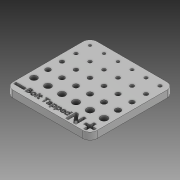
# Autodesk Inventor part: Tapped Test Print
Saved by Autodesk Inventor 2022 (Build 260153000, 153)
## iProperties
Created: 2022-01-18
Part Number: Tapped Test Print
Material: ABS Plastic
Document SubType Name: Modeling
Density: 1.06 g/cm^3
Appearance: Smooth - Medium Gray
Autodesk Inventor part; units mm, degrees
ref_plane "YZ Plane" through (0, 0, 0) normal (1, 0, 0) x (0, 1, 0)
ref_plane "XZ Plane" through (0, 0, 0) normal (0, 1, 0) x (-1, 0, 0)
ref_plane "XY Plane" through (0, 0, 0) normal (0, 0, 1) x (1, 0, 0)
sketch "Sketch1" plane through (0, 0, 0) normal (0, 1, 0) x (-1, 0, 0)
  circle A0 centre (0, 12.7) radius 1.4986
  circle A1 centre (-12.7, 12.7) radius 1.5621
  circle A2 centre (-25.4, 12.7) radius 1.6256
  circle A3 centre (-38.1, 12.7) radius 1.6891
  circle A4 centre (-50.8, 12.7) radius 1.7526
  circle A5 centre (0, 25.4) radius 1.8288
  circle A6 centre (-12.7, 25.4) radius 1.8923
  circle A7 centre (-25.4, 25.4) radius 1.9558
  circle A8 centre (-38.1, 25.4) radius 2.0193
  circle A9 centre (-50.8, 25.4) radius 2.0828
  circle A10 centre (0, 38.1) radius 2.2352
  circle A11 centre (-12.7, 38.1) radius 2.2987
  circle A12 centre (-25.4, 38.1) radius 2.3622
  circle A13 centre (-38.1, 38.1) radius 2.4257
  circle A14 centre (-50.8, 38.1) radius 2.4892
  line L0 (4.7625, 64.6906) -> (-4.7625, 64.6906)
  line L1 (-4.7625, 64.6906) -> (-4.7625, 62.3094)
  line L2 (-4.7625, 62.3094) -> (4.7625, 62.3094)
  line L3 (4.7625, 62.3094) -> (4.7625, 64.6906)
  line L4 (4.7625, 64.6906) -> (-4.7625, 62.3094) construction
  line L5 (-4.7625, 64.6906) -> (4.7625, 62.3094) construction
  line L6 (-58.7375, 64.6906) -> (-68.2625, 64.6906)
  line L7 (-68.2625, 64.6906) -> (-68.2625, 62.3094)
  line L8 (-68.2625, 62.3094) -> (-58.7375, 62.3094)
  line L9 (-58.7375, 62.3094) -> (-58.7375, 64.6906)
  line L10 (-58.7375, 64.6906) -> (-68.2625, 62.3094) construction
  line L11 (-68.2625, 64.6906) -> (-58.7375, 62.3094) construction
  line L12 (-64.6906, 58.7375) -> (-62.3094, 58.7375)
  line L13 (-62.3094, 58.7375) -> (-62.3094, 68.2625)
  line L14 (-62.3094, 68.2625) -> (-64.6906, 68.2625)
  line L15 (-64.6906, 68.2625) -> (-64.6906, 58.7375)
  line L16 (-64.6906, 58.7375) -> (-62.3094, 68.2625) construction
  line L17 (-62.3094, 58.7375) -> (-64.6906, 68.2625) construction
  circle A15 centre (-63.5, 38.1) radius 2.5527
  circle A16 centre (-63.5, 25.4) radius 2.1463
  circle A17 centre (-63.5, 12.7) radius 1.8161
  circle A18 centre (0, 0) radius 1.1684
  circle A19 centre (-12.7, 0) radius 1.2319
  circle A20 centre (-25.4, 0) radius 1.2954
  circle A21 centre (-38.1, 0) radius 1.3589
  circle A22 centre (-50.8, 0) radius 1.4224
  circle A23 centre (-63.5, 0) radius 1.4859
  line L18 (-46.0375, 68.2625) -> (-46.0375, 58.7375)
  line L19 (-46.0375, 58.7375) -> (-48.4188, 58.7375)
  line L20 (-48.4188, 58.7375) -> (-53.1813, 64.5177)
  line L21 (-53.1813, 64.5177) -> (-53.1813, 58.7375)
  line L22 (-53.1813, 58.7375) -> (-55.5625, 58.7375)
  line L23 (-55.5625, 58.7375) -> (-55.5625, 68.2625)
  line L24 (-55.5625, 68.2625) -> (-53.1813, 68.2625)
  line L25 (-53.1813, 68.2625) -> (-48.4188, 62.4823)
  line L26 (-48.4188, 62.4823) -> (-48.4188, 68.2625)
  line L27 (-48.4188, 68.2625) -> (-46.0375, 68.2625)
  line L28 (-50.8, 65.3724) -> (-50.8, 61.6276) construction
  line L29 (6.35, -6.35) -> (-69.85, -6.35)
  line L30 (-69.85, -6.35) -> (-69.85, 69.85)
  line L31 (-69.85, 69.85) -> (6.35, 69.85)
  line L32 (6.35, 69.85) -> (6.35, -6.35)
  line L33 (6.35, -6.35) -> (-69.85, 69.85) construction
  line L34 (-69.85, -6.35) -> (6.35, 69.85) construction
  circle A24 centre (-12.7, 50.8) radius 2.9845
  circle A25 centre (-25.4, 50.8) radius 3.048
  circle A26 centre (-38.1, 50.8) radius 3.1115
  circle A27 centre (-50.8, 50.8) radius 3.175
  circle A28 centre (-63.5, 50.8) radius 3.2385
  circle A29 centre (0, 50.8) radius 2.921
  line L35 (0, 73.2249) -> (-50.8, 73.2249) construction
  line L36 (-50.8, 73.2249) -> (-50.8, 53.7751) construction
  line L37 (-50.8, 53.7751) -> (0, 53.7751) construction
  line L38 (0, 53.7751) -> (0, 73.2249) construction
  spline S0 degree 2 poles (-9.9909, 63.8715) (-9.9909, 64.2275) (-9.72, 64.7654) (-9.4956, 64.9434) knots 0 0 0 1 2 2 2
  spline S1 degree 2 poles (-9.4956, 64.9434) (-9.2247, 65.1562) (-8.5823, 65.3342) (-8.0831, 65.3342) knots 0 0 0 1 2 2 2
  line L39 (-8.0831, 65.3342) -> (-6.1754, 65.3342)
  line L40 (-6.1754, 65.3342) -> (-6.1754, 60.559)
  line L41 (-6.1754, 60.559) -> (-7.8587, 60.559)
  spline S2 degree 2 poles (-7.8587, 60.559) (-8.385, 60.559) (-8.9267, 60.6403) (-9.1628, 60.768) knots 0 0 0 1 2 2 2
  spline S3 degree 2 poles (-9.1628, 60.768) (-9.422, 60.9034) (-9.6736, 61.3678) (-9.6736, 61.6696) knots 0 0 0 1 2 2 2
  spline S4 degree 2 poles (-9.6736, 61.6696) (-9.6736, 62.0179) (-9.3253, 62.5635) (-9.0157, 62.6912) knots 0 0 0 1 2 2 2
  line L42 (-9.0157, 62.6912) -> (-9.0157, 62.7145)
  spline S5 degree 2 poles (-9.0157, 62.7145) (-9.4607, 62.8073) (-9.9909, 63.3839) (-9.9909, 63.8715) knots 0 0 0 1 2 2 2
  spline S6 degree 2 poles (-8.7526, 63.8521) (-8.7526, 63.6277) (-8.5746, 63.3762) (-8.3966, 63.3104) knots 0 0 0 1 2 2 2
  spline S7 degree 2 poles (-8.3966, 63.3104) (-8.2882, 63.2678) (-7.9051, 63.2601) (-7.5878, 63.2601) knots 0 0 0 1 2 2 2
  line L43 (-7.5878, 63.2601) -> (-7.3672, 63.2601)
  line L44 (-7.3672, 63.2601) -> (-7.3672, 64.4636)
  line L45 (-7.3672, 64.4636) -> (-7.433, 64.4636)
  spline S8 degree 2 poles (-7.433, 64.4636) (-7.8974, 64.4636) (-8.2534, 64.4519) (-8.4391, 64.3707) knots 0 0 0 1 2 2 2
  spline S9 degree 2 poles (-8.4391, 64.3707) (-8.6017, 64.2972) (-8.7526, 64.0263) (-8.7526, 63.8521) knots 0 0 0 1 2 2 2
  spline S10 degree 2 poles (-8.4546, 61.9057) (-8.4546, 61.7896) (-8.3347, 61.5458) (-8.2108, 61.4916) knots 0 0 0 1 2 2 2
  spline S11 degree 2 poles (-8.2108, 61.4916) (-8.0947, 61.4375) (-7.7697, 61.4297) (-7.4485, 61.4297) knots 0 0 0 1 2 2 2
  line L46 (-7.4485, 61.4297) -> (-7.3672, 61.4297)
  line L47 (-7.3672, 61.4297) -> (-7.3672, 62.4436)
  line L48 (-7.3672, 62.4436) -> (-7.5182, 62.4436)
  spline S12 degree 2 poles (-7.5182, 62.4436) (-7.8239, 62.4436) (-8.0715, 62.432) (-8.2031, 62.37) knots 0 0 0 1 2 2 2
  spline S13 degree 2 poles (-8.2031, 62.37) (-8.3463, 62.3004) (-8.4546, 62.0643) (-8.4546, 61.9057) knots 0 0 0 1 2 2 2
  spline S14 degree 2 poles (-14.0695, 63.5348) (-14.0695, 64.4249) (-13.0982, 65.4465) (-12.2121, 65.4465) knots 0 0 0 1 2 2 2
  spline S15 degree 2 poles (-12.2121, 65.4465) (-11.3298, 65.4465) (-10.3508, 64.4249) (-10.3508, 63.5348) knots 0 0 0 1 2 2 2
  spline S16 degree 2 poles (-10.3508, 63.5348) (-10.3508, 62.6371) (-11.3298, 61.6193) (-12.2121, 61.6193) knots 0 0 0 1 2 2 2
  spline S17 degree 2 poles (-12.2121, 61.6193) (-13.0944, 61.6193) (-14.0695, 62.6409) (-14.0695, 63.5348) knots 0 0 0 1 2 2 2
  spline S18 degree 2 poles (-12.9202, 63.5426) (-12.9202, 63.2214) (-12.8158, 62.7918) (-12.7229, 62.6641) knots 0 0 0 1 2 2 2
  spline S19 degree 2 poles (-12.7229, 62.6641) (-12.6223, 62.5287) (-12.3707, 62.4242) (-12.2121, 62.4242) knots 0 0 0 1 2 2 2
  spline S20 degree 2 poles (-12.2121, 62.4242) (-12.0573, 62.4242) (-11.8135, 62.5171) (-11.7129, 62.6487) knots 0 0 0 1 2 2 2
  spline S21 degree 2 poles (-11.7129, 62.6487) (-11.6162, 62.7725) (-11.5001, 63.2098) (-11.5001, 63.5426) knots 0 0 0 1 2 2 2
  spline S22 degree 2 poles (-11.5001, 63.5426) (-11.5001, 63.8715) (-11.6084, 64.2778) (-11.6974, 64.4016) knots 0 0 0 1 2 2 2
  spline S23 degree 2 poles (-11.6974, 64.4016) (-11.7864, 64.5255) (-12.0573, 64.6416) (-12.2198, 64.6416) knots 0 0 0 1 2 2 2
  spline S24 degree 2 poles (-12.2198, 64.6416) (-12.3553, 64.6416) (-12.6339, 64.5255) (-12.719, 64.4094) knots 0 0 0 1 2 2 2
  spline S25 degree 2 poles (-12.719, 64.4094) (-12.8158, 64.2739) (-12.9202, 63.8831) (-12.9202, 63.5426) knots 0 0 0 1 2 2 2
  line L49 (-15.7877, 65.3342) -> (-14.6655, 65.3342)
  line L50 (-14.6655, 65.3342) -> (-14.6655, 60.3462)
  line L51 (-14.6655, 60.3462) -> (-15.7877, 60.3462)
  line L52 (-15.7877, 60.3462) -> (-15.7877, 65.3342)
  spline S26 degree 2 poles (-18.0244, 65.4039) (-17.3394, 65.4039) (-16.7125, 64.8389) (-16.7125, 64.1965) knots 0 0 0 1 2 2 2
  line L53 (-16.7125, 64.1965) -> (-16.7125, 62.5132)
  line L54 (-16.7125, 62.5132) -> (-16.283, 62.5132)
  line L55 (-16.283, 62.5132) -> (-16.283, 61.7316)
  line L56 (-16.283, 61.7316) -> (-16.7125, 61.7316)
  line L57 (-16.7125, 61.7316) -> (-16.7125, 60.7022)
  line L58 (-16.7125, 60.7022) -> (-17.8348, 60.7022)
  line L59 (-17.8348, 60.7022) -> (-17.8348, 61.7316)
  line L60 (-17.8348, 61.7316) -> (-18.9183, 61.7316)
  line L61 (-18.9183, 61.7316) -> (-18.9183, 62.5132)
  line L62 (-18.9183, 62.5132) -> (-17.8348, 62.5132)
  line L63 (-17.8348, 62.5132) -> (-17.8348, 63.7941)
  spline S27 degree 2 poles (-17.8348, 63.7941) (-17.8348, 63.9837) (-17.8425, 64.2662) (-17.8889, 64.3784) knots 0 0 0 1 2 2 2
  spline S28 degree 2 poles (-17.8889, 64.3784) (-17.9354, 64.4906) (-18.1637, 64.6222) (-18.3804, 64.6222) knots 0 0 0 1 2 2 2
  spline S29 degree 2 poles (-18.3804, 64.6222) (-18.4733, 64.6222) (-18.7635, 64.5448) (-18.8215, 64.5139) knots 0 0 0 1 2 2 2
  line L64 (-18.8215, 64.5139) -> (-18.9183, 64.5139)
  line L65 (-18.9183, 64.5139) -> (-18.9183, 65.3033)
  spline S30 degree 2 poles (-18.9183, 65.3033) (-18.7364, 65.3497) (-18.3262, 65.4039) (-18.0244, 65.4039) knots 0 0 0 1 2 2 2
  line L66 (-22.281, 65.3342) -> (-22.281, 61.4684)
  line L67 (-22.281, 61.4684) -> (-20.8686, 61.4684)
  line L68 (-20.8686, 61.4684) -> (-20.8686, 60.559)
  line L69 (-20.8686, 60.559) -> (-24.8931, 60.559)
  line L70 (-24.8931, 60.559) -> (-24.8931, 61.4684)
  line L71 (-24.8931, 61.4684) -> (-23.4806, 61.4684)
  line L72 (-23.4806, 61.4684) -> (-23.4806, 65.3342)
  line L73 (-23.4806, 65.3342) -> (-22.281, 65.3342)
  spline S31 degree 2 poles (-27.3039, 64.9511) (-27.1878, 65.0479) (-27.0059, 65.2027) (-26.8511, 65.2801) knots 0 0 0 1 2 2 2
  spline S32 degree 2 poles (-26.8511, 65.2801) (-26.7002, 65.3536) (-26.4139, 65.431) (-26.1585, 65.431) knots 0 0 0 1 2 2 2
  spline S33 degree 2 poles (-26.1585, 65.431) (-25.6786, 65.431) (-25.0479, 64.7886) (-25.0479, 64.301) knots 0 0 0 1 2 2 2
  spline S34 degree 2 poles (-25.0479, 64.301) (-25.0479, 63.9024) (-25.369, 63.4071) (-25.6709, 63.2639) knots 0 0 0 1 2 2 2
  spline S35 degree 2 poles (-25.6709, 63.2639) (-25.9766, 63.1169) (-26.824, 63.0008) (-27.3116, 62.9699) knots 0 0 0 1 2 2 2
  line L74 (-27.3116, 62.9699) -> (-27.3116, 62.9505)
  spline S36 degree 2 poles (-27.3116, 62.9505) (-27.3116, 62.6525) (-26.8705, 62.4242) (-26.4293, 62.4242) knots 0 0 0 1 2 2 2
  spline S37 degree 2 poles (-26.4293, 62.4242) (-26.232, 62.4242) (-25.698, 62.5674) (-25.4464, 62.6796) knots 0 0 0 1 2 2 2
  line L75 (-25.4464, 62.6796) -> (-25.3497, 62.6796)
  line L76 (-25.3497, 62.6796) -> (-25.3497, 61.8089)
  spline S38 degree 2 poles (-25.3497, 61.8089) (-25.5161, 61.7625) (-26.2591, 61.6309) (-26.6383, 61.6309) knots 0 0 0 1 2 2 2
  spline S39 degree 2 poles (-26.6383, 61.6309) (-27.567, 61.6309) (-28.4184, 62.2501) (-28.4184, 62.8847) knots 0 0 0 1 2 2 2
  line L77 (-28.4184, 62.8847) -> (-28.4184, 65.3342)
  line L78 (-28.4184, 65.3342) -> (-27.3039, 65.3342)
  line L79 (-27.3039, 65.3342) -> (-27.3039, 64.9511)
  line L80 (-27.3039, 64.3939) -> (-27.3039, 63.647)
  spline S40 degree 2 poles (-27.3039, 63.647) (-27.0175, 63.6741) (-26.6654, 63.7167) (-26.4951, 63.7786) knots 0 0 0 1 2 2 2
  spline S41 degree 2 poles (-26.4951, 63.7786) (-26.3442, 63.8289) (-26.1817, 64.0379) (-26.1817, 64.2082) knots 0 0 0 1 2 2 2
  spline S42 degree 2 poles (-26.1817, 64.2082) (-26.1817, 64.4597) (-26.4564, 64.6493) (-26.7234, 64.6493) knots 0 0 0 1 2 2 2
  spline S43 degree 2 poles (-26.7234, 64.6493) (-26.8705, 64.6493) (-27.1801, 64.5139) (-27.3039, 64.3939) knots 0 0 0 1 2 2 2
  spline S44 degree 2 poles (-32.7795, 63.4845) (-32.7795, 64.3475) (-31.905, 65.4039) (-31.2626, 65.4039) knots 0 0 0 1 2 2 2
  spline S45 degree 2 poles (-31.2626, 65.4039) (-30.9956, 65.4039) (-30.597, 65.2839) (-30.3726, 65.1524) knots 0 0 0 1 2 2 2
  line L81 (-30.3726, 65.1524) -> (-30.3726, 66.6538)
  line L82 (-30.3726, 66.6538) -> (-29.2503, 66.6538)
  line L83 (-29.2503, 66.6538) -> (-29.2503, 61.7316)
  line L84 (-29.2503, 61.7316) -> (-30.3726, 61.7316)
  line L85 (-30.3726, 61.7316) -> (-30.3726, 62.1108)
  spline S46 degree 2 poles (-30.3726, 62.1108) (-30.6202, 61.8979) (-31.131, 61.6348) (-31.4677, 61.6348) knots 0 0 0 1 2 2 2
  spline S47 degree 2 poles (-31.4677, 61.6348) (-32.0946, 61.6348) (-32.7795, 62.6293) (-32.7795, 63.4845) knots 0 0 0 1 2 2 2
  spline S48 degree 2 poles (-31.6302, 63.5077) (-31.6302, 62.9815) (-31.3052, 62.5094) (-30.9646, 62.5094) knots 0 0 0 1 2 2 2
  spline S49 degree 2 poles (-30.9646, 62.5094) (-30.8137, 62.5094) (-30.5157, 62.6061) (-30.3726, 62.7028) knots 0 0 0 1 2 2 2
  line L86 (-30.3726, 62.7028) -> (-30.3726, 64.51)
  spline S50 degree 2 poles (-30.3726, 64.51) (-30.4616, 64.5487) (-30.6783, 64.5796) (-30.8253, 64.5796) knots 0 0 0 1 2 2 2
  spline S51 degree 2 poles (-30.8253, 64.5796) (-31.2316, 64.5796) (-31.6302, 64.0456) (-31.6302, 63.5077) knots 0 0 0 1 2 2 2
  spline S52 degree 2 poles (-36.9123, 63.4845) (-36.9123, 64.3475) (-36.0378, 65.4039) (-35.3954, 65.4039) knots 0 0 0 1 2 2 2
  spline S53 degree 2 poles (-35.3954, 65.4039) (-35.1284, 65.4039) (-34.7298, 65.2839) (-34.5054, 65.1524) knots 0 0 0 1 2 2 2
  line L87 (-34.5054, 65.1524) -> (-34.5054, 66.6538)
  line L88 (-34.5054, 66.6538) -> (-33.3832, 66.6538)
  line L89 (-33.3832, 66.6538) -> (-33.3832, 61.7316)
  line L90 (-33.3832, 61.7316) -> (-34.5054, 61.7316)
  line L91 (-34.5054, 61.7316) -> (-34.5054, 62.1108)
  spline S54 degree 2 poles (-34.5054, 62.1108) (-34.753, 61.8979) (-35.2638, 61.6348) (-35.6005, 61.6348) knots 0 0 0 1 2 2 2
  spline S55 degree 2 poles (-35.6005, 61.6348) (-36.2274, 61.6348) (-36.9123, 62.6293) (-36.9123, 63.4845) knots 0 0 0 1 2 2 2
  spline S56 degree 2 poles (-35.763, 63.5077) (-35.763, 62.9815) (-35.438, 62.5094) (-35.0974, 62.5094) knots 0 0 0 1 2 2 2
  spline S57 degree 2 poles (-35.0974, 62.5094) (-34.9465, 62.5094) (-34.6486, 62.6061) (-34.5054, 62.7028) knots 0 0 0 1 2 2 2
  line L92 (-34.5054, 62.7028) -> (-34.5054, 64.51)
  spline S58 degree 2 poles (-34.5054, 64.51) (-34.5944, 64.5487) (-34.8111, 64.5796) (-34.9581, 64.5796) knots 0 0 0 1 2 2 2
  spline S59 degree 2 poles (-34.9581, 64.5796) (-35.3645, 64.5796) (-35.763, 64.0456) (-35.763, 63.5077) knots 0 0 0 1 2 2 2
  spline S60 degree 2 poles (-39.3618, 65.431) (-38.3403, 65.431) (-37.2529, 64.4558) (-37.2529, 63.5542) knots 0 0 0 1 2 2 2
  spline S61 degree 2 poles (-37.2529, 63.5542) (-37.2529, 62.6719) (-38.2667, 61.6193) (-39.18, 61.6193) knots 0 0 0 1 2 2 2
  spline S62 degree 2 poles (-39.18, 61.6193) (-40.0042, 61.6193) (-40.8401, 62.5132) (-40.8401, 63.3413) knots 0 0 0 1 2 2 2
  line L93 (-40.8401, 63.3413) -> (-40.8401, 63.7477)
  line L94 (-40.8401, 63.7477) -> (-38.3751, 63.7477)
  spline S63 degree 2 poles (-38.3751, 63.7477) (-38.3906, 63.9992) (-38.5724, 64.332) (-38.7195, 64.4326) knots 0 0 0 1 2 2 2
  spline S64 degree 2 poles (-38.7195, 64.4326) (-38.8627, 64.5332) (-39.2496, 64.6183) (-39.4779, 64.6183) knots 0 0 0 1 2 2 2
  spline S65 degree 2 poles (-39.4779, 64.6183) (-39.6714, 64.6183) (-40.0507, 64.5332) (-40.2093, 64.4597) knots 0 0 0 1 2 2 2
  spline S66 degree 2 poles (-40.2093, 64.4597) (-40.3486, 64.4016) (-40.5808, 64.2585) (-40.6543, 64.2043) knots 0 0 0 1 2 2 2
  line L95 (-40.6543, 64.2043) -> (-40.7743, 64.2043)
  line L96 (-40.7743, 64.2043) -> (-40.7743, 65.133)
  spline S67 degree 2 poles (-40.7743, 65.133) (-40.635, 65.1872) (-40.4105, 65.2801) (-40.2093, 65.3265) knots 0 0 0 1 2 2 2
  spline S68 degree 2 poles (-40.2093, 65.3265) (-40.0274, 65.3768) (-39.6405, 65.431) (-39.3618, 65.431) knots 0 0 0 1 2 2 2
  spline S69 degree 2 poles (-39.7333, 63.0705) (-39.7256, 62.7145) (-39.4122, 62.3391) (-39.091, 62.3391) knots 0 0 0 1 2 2 2
  spline S70 degree 2 poles (-39.091, 62.3391) (-38.762, 62.3391) (-38.3906, 62.7338) (-38.3712, 63.0705) knots 0 0 0 1 2 2 2
  line L97 (-38.3712, 63.0705) -> (-39.7333, 63.0705)
  line L98 (-44.6904, 65.3342) -> (-43.5682, 65.3342)
  line L99 (-43.5682, 65.3342) -> (-43.5682, 64.9589)
  spline S71 degree 2 poles (-43.5682, 64.9589) (-43.4599, 65.0479) (-43.1812, 65.253) (-43.0729, 65.3071) knots 0 0 0 1 2 2 2
  spline S72 degree 2 poles (-43.0729, 65.3071) (-42.9413, 65.3691) (-42.6782, 65.4348) (-42.4963, 65.4348) knots 0 0 0 1 2 2 2
  spline S73 degree 2 poles (-42.4963, 65.4348) (-41.881, 65.4348) (-41.1613, 64.4132) (-41.1613, 63.5619) knots 0 0 0 1 2 2 2
  spline S74 degree 2 poles (-41.1613, 63.5619) (-41.1613, 63.0898) (-41.405, 62.3971) (-41.6179, 62.1417) knots 0 0 0 1 2 2 2
  spline S75 degree 2 poles (-41.6179, 62.1417) (-41.8152, 61.9057) (-42.3725, 61.6348) (-42.682, 61.6348) knots 0 0 0 1 2 2 2
  spline S76 degree 2 poles (-42.682, 61.6348) (-42.9645, 61.6348) (-43.3283, 61.7548) (-43.5682, 61.8786) knots 0 0 0 1 2 2 2
  line L100 (-43.5682, 61.8786) -> (-43.5682, 60.3462)
  line L101 (-43.5682, 60.3462) -> (-44.6904, 60.3462)
  line L102 (-44.6904, 60.3462) -> (-44.6904, 65.3342)
  line L103 (-43.5682, 64.3436) -> (-43.5682, 62.5751)
  spline S77 degree 2 poles (-43.5682, 62.5751) (-43.4869, 62.5326) (-43.2161, 62.4784) (-43.1193, 62.4784) knots 0 0 0 1 2 2 2
  spline S78 degree 2 poles (-43.1193, 62.4784) (-42.7169, 62.4784) (-42.3106, 63.0434) (-42.3106, 63.5503) knots 0 0 0 1 2 2 2
  spline S79 degree 2 poles (-42.3106, 63.5503) (-42.3106, 64.0843) (-42.6356, 64.5603) (-42.9955, 64.5603) knots 0 0 0 1 2 2 2
  spline S80 degree 2 poles (-42.9955, 64.5603) (-43.1425, 64.5603) (-43.4444, 64.4442) (-43.5682, 64.3436) knots 0 0 0 1 2 2 2
  point P0 (0, 63.5)
  point P1 (-63.5, 63.5)
  point P2 (-63.5, 63.5)
  point P3 (0, 63.5)
  point P4 (-63.5, 63.5)
  point P5 (0, 63.5)
  point P6 (-63.5, 63.5)
  point P7 (-64.6906, 64.6906)
  point P8 (-62.3094, 64.6906)
  point P9 (-62.3094, 62.3094)
  point P10 (-64.6906, 62.3094)
  point P11 (-50.8, 63.5)
  point P12 (-63.5, 63.5)
  point P13 (-31.75, 31.75)
  point P14 (-31.75, 31.75)
  point P15 (-25.4, 53.7751)
  point P16 (0, 63.5)
  dimension "d1" = 2.9972
  dimension "d2" = 3.1242
  dimension "d3" = 3.2512
  dimension "d4" = 3.3782
  dimension "d5" = 3.5052
  dimension "d6" = 3.6576
  dimension "d7" = 3.7846
  dimension "d8" = 3.9116
  dimension "d9" = 4.0386
  dimension "d10" = 4.1656
  dimension "d11" = 4.4704
  dimension "d12" = 4.5974
  dimension "d13" = 4.7244
  dimension "d14" = 4.8514
  dimension "d15" = 4.9784
  dimension "d33" = 9.525
  dimension "d34" = 2.3813
  dimension "d43" = 3.6322
  dimension "d44" = 4.2926
  dimension "d45" = 5.1054
  dimension "d47" = 2.4638
  dimension "d48" = 2.3368
  dimension "d49" = 2.5908
  dimension "d50" = 2.7178
  dimension "d51" = 2.8448
  dimension "d52" = 2.9718
  dimension "d53" = 12.7
  dimension "d54" = 12.7
  dimension "d55" = 12.7
  dimension "d56" = 12.7
  dimension "d57" = 12.7
  dimension "d58" = 12.7
  dimension "d59" = 12.7
  dimension "d60" = 12.7
  dimension "d61" = 9.525
  dimension "d62" = 9.525
  dimension "d64" = 2.3813
  dimension "d66" = 76.2
  dimension "d67" = 76.2
  dimension "d69" = 6.35
  dimension "d70" = 6.35
  dimension "d71" = 5.969
  dimension "d72" = 6.096
  dimension "d73" = 6.223
  dimension "d74" = 6.35
  dimension "d75" = 6.477
  dimension "d76" = 5.842
  dimension "d77" = 12.7
  dimension "d78" = 12.7
  constraints: 71 end point, 30 centre point, 28 vertical alignment, 27 horizontal alignment, 20 midpoint, 11 parallel, 7 equal length, 7 perpendicular, 6 point on line, 4 horizontal, 3 coincident, 2 vertical, 2 other
  measures "d1" diameter of A0
  measures "d2" diameter of A1
  measures "d3" diameter of A2
  measures "d4" diameter of A3
  measures "d5" diameter of A4
  measures "d6" diameter of A5
  measures "d7" diameter of A6
  measures "d8" diameter of A7
  measures "d9" diameter of A8
  measures "d10" diameter of A9
  measures "d11" diameter of A10
  measures "d12" diameter of A11
  measures "d13" diameter of A12
  measures "d14" diameter of A13
  measures "d15" diameter of A14
  measures "d33" distance of L1.end L2.end
  measures "d34" distance of L2.end L0.start
  measures "d43" diameter of A17
  measures "d44" diameter of A16
  measures "d45" diameter of A15
  measures "d47" diameter of A19
  measures "d48" diameter of A18
  measures "d49" diameter of A20
  measures "d50" diameter of A21
  measures "d51" diameter of A22
  measures "d52" diameter of A23
  measures "d53" distance of A19.centre A18.centre
  measures "d54" distance of A20.centre A19.centre
  measures "d55" distance of A21.centre A20.centre
  measures "d56" distance of A22.centre A21.centre
  measures "d57" distance of A23.centre A22.centre
  measures "d58" distance of point (0, 12.7) A18.centre
  measures "d59" distance of A5.centre point (0, 12.7)
  measures "d60" distance of A10.centre A5.centre
  measures "d61" distance between parallel lines of L23 L18
  measures "d62" distance between parallel lines of L24 L22
  measures "d64" distance between parallel lines of L25 L20
  measures "d66" distance of L29.end L30.end
  measures "d67" distance of L29.start L29.end
  measures "d69" horizontal distance of point (-31.75, 31.75) A7.centre
  measures "d70" horizontal distance of point (-31.75, 31.75) A7.centre
  measures "d71" diameter of A24
  measures "d72" diameter of A25
  measures "d73" diameter of A26
  measures "d74" diameter of A27
  measures "d75" diameter of A28
  measures "d76" diameter of A29
  measures "d77" distance of A29.centre A10.centre
  measures "d78" distance of A29.centre point (0, 63.5)
extrude "Extrusion1" add sketch "Sketch1" against normal blind 6.35 contours L29 L30 L31 L32 | S0 S1 L39 L40 L41 S2 S3 S4 L42 S5 | S9 S8 L45 L44 L43 S7 S6 | S13 S12 L48 L47 L46 S11 S10 | S14 S15 S16 S17 | S25 S24 S23 S22 S21 S20 S19 S18 | L49 L50 L51 L52 | S26 L53 L54 L55 L56 L57 L58 L59 L60 L61 L62 L63 S27 S28 S29 L64 L65 S30 | L66 L67 L68 L69 L70 L71 L72 L73 | S31 S32 S33 S34 S35 L74 S36 S37 L75 L76 S38 S39 L77 L78 L79 | S43 S42 S41 S40 L80 | S44 S45 L81 L82 L83 L84 L85 S46 S47 | S51 S50 L86 S49 S48 | S52 S53 L87 L88 L89 L90 L91 S54 S55 | S59 S58 L92 S57 S56 | S60 S61 S62 L93 L94 S63 S64 S65 S66 L95 L96 S67 S68 | L97 S70 S69 | L98 L99 S71 S72 S73 S74 S75 S76 L100 L101 L102 | S80 S79 S78 S77 L103
fillet "Fillet1" radius 6.35 4 edges at (-6.35, -3.175, 69.85) (-6.35, -3.175, -6.35) (69.85, -3.175, -6.35) (69.85, -3.175, 69.85)
fillet "Fillet2" radius 0.3969 26 edges at (53.1813, -3.175, 64.5177) (68.2625, -3.175, 62.3094) (68.2625, -3.175, 64.6906) (64.6906, -3.175, 64.6906) (64.6906, -3.175, 68.2625) (62.3094, -3.175, 68.2625) (62.3094, -3.175, 64.6906) (58.7375, -3.175, 64.6906) (58.7375, -3.175, 62.3094) (62.3094, -3.175, 62.3094) (62.3094, -3.175, 58.7375) (64.6906, -3.175, 58.7375) (64.6906, -3.175, 62.3094) (53.1813, -3.175, 58.7375) (55.5625, -3.175, 58.7375) (55.5625, -3.175, 68.2625) (53.1813, -3.175, 68.2625) (48.4188, -3.175, 62.4823) (48.4188, -3.175, 58.7375) (46.0375, -3.175, 58.7375) (48.4188, -3.175, 68.2625) (46.0375, -3.175, 68.2625) (4.7625, -3.175, 64.6906) (4.7625, -3.175, 62.3094) (-4.7625, -3.175, 62.3094) (-4.7625, -3.175, 64.6906)
emboss "Emboss1" sketch "Sketch1" operation cut depth 3.175 direction (0, -1, 0) contours S0 S1 L39 L40 L41 S2 S3 S4 L42 S5 | S14 S15 S16 S17 | L49 L50 L51 L52 | S26 L53 L54 L55 L56 L57 L58 L59 L60 L61 L62 L63 S27 S28 S29 L64 L65 S30 | L66 L67 L68 L69 L70 L71 L72 L73 | S31 S32 S33 S34 S35 L74 S36 S37 L75 L76 S38 S39 L77 L78 L79 | S44 S45 L81 L82 L83 L84 L85 S46 S47 | S52 S53 L87 L88 L89 L90 L91 S54 S55 | S60 S61 S62 L93 L94 S63 S64 S65 S66 L95 L96 S67 S68 | L98 L99 S71 S72 S73 S74 S75 S76 L100 L101 L102
body "Solid1"
